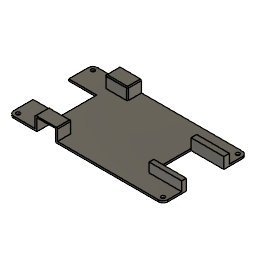
BASE (Autodesk Fusion 360 design; units mm, degrees)
Autodesk Fusion 360 part; units mm, degrees
sketch "Sketch1" plane through (0, 0, 0) normal (0, 0, 1) x (1, 0, 0)
  line L0 (0, 0) -> (165, 0)
  line L1 (165, 0) -> (165, 90)
  line L2 (165, 90) -> (0, 90)
  line L3 (0, 90) -> (0, 0)
  dimension "d1" = 165
  dimension "d2" = 90
  constraint horizontal L0
  constraint vertical L1
  constraint horizontal L2
  constraint vertical L3
  constraint coincident L0.start L3.end
  measures "d1" distance of L0.start L0.end
  measures "d2" distance of L0.start L2.end
extrude "Extrude1" add sketch "Sketch1" along normal blind 3
fillet "Fillet1" radius 5 1 edges at (0, 0, 1.5)
fillet "Fillet1" radius 5 3 edges at (0, 90, 1.5) (165, 90, 1.5) (165, 0, 1.5)
sketch "Sketch4" plane through (0, 0, 3) normal (0, 0, 1) x (-1, 0, 0)
  arc A0 (-160, 0) -> (-165, -5) centre (-160, -5) ccw
  line L0 (-165, -5) -> (-165, -85)
  arc A1 (-165, -85) -> (-160, -90) centre (-160, -85) ccw
  line L1 (-160, -90) -> (-5, -90)
  arc A2 (-5, -90) -> (0, -85) centre (-5, -85) ccw
  line L2 (0, -85) -> (0, -5)
  arc A3 (0, -5) -> (-5, 0) centre (-5, -5) ccw
  line L3 (-5, 0) -> (-160, 0)
  line L4 (-30, -90) -> (-50, -90)
  line L5 (-50, -90) -> (-50, -77)
  line L6 (-50, -77) -> (-30, -77)
  line L7 (-30, -77) -> (-30, -90)
  line L8 (-30, 0) -> (-50, 0)
  line L9 (-50, 0) -> (-50, -13)
  line L10 (-50, -13) -> (-30, -13)
  line L11 (-30, -13) -> (-30, 0)
  dimension "d9" = 20
  dimension "d10" = 13
  dimension "d11" = 20
  dimension "d12" = 13
  constraint horizontal L4
  constraint vertical L5
  constraint horizontal L6
  constraint vertical L7
  constraint coincident L1 L4.start
  constraint horizontal L8
  constraint vertical L9
  constraint horizontal L10
  constraint vertical L11
  constraint coincident L3 L8.start
  measures "d9" distance of L4.start L4.end
  measures "d10" distance of L4.start L6.end
  measures "d11" distance of L8.start L8.end
  measures "d12" distance of L8.start L10.end
extrude "Extrude2" cut sketch "Sketch4" against normal blind 3 contours L3 L8 L9 L10 L11 | L1 L4 L5 L6 L7
sketch "Sketch5" plane through (0, 0, 3) normal (0, 0, 1) x (-1, 0, 0)
  line L0 (-30, -77) -> (-30, -90)
  line L1 (-30, -90) -> (-5, -90)
  arc A0 (-5, -90) -> (0, -85) centre (-5, -85) ccw
  line L2 (0, -85) -> (0, -5)
  arc A1 (0, -5) -> (-5, 0) centre (-5, -5) ccw
  line L3 (-5, 0) -> (-30, 0)
  line L4 (-30, 0) -> (-30, -13)
  line L5 (-30, -13) -> (-50, -13)
  line L6 (-50, -13) -> (-50, 0)
  line L7 (-50, 0) -> (-160, 0)
  arc A2 (-160, 0) -> (-165, -5) centre (-160, -5) ccw
  line L8 (-165, -5) -> (-165, -85)
  arc A3 (-165, -85) -> (-160, -90) centre (-160, -85) ccw
  line L9 (-160, -90) -> (-50, -90)
  line L10 (-50, -90) -> (-50, -77)
  line L11 (-50, -77) -> (-30, -77)
  circle A4 centre (-120, -45) radius 35
  dimension "d41" = 70
  measures "d41" diameter of A4
sketch "Sketch6" plane through (0, 0, 3) normal (0, 0, 1) x (-1, 0, 0)
  line L0 (-30, -77) -> (-30, -90)
  line L1 (-30, -90) -> (-5, -90)
  arc A0 (-5, -90) -> (0, -85) centre (-5, -85) ccw
  line L2 (0, -85) -> (0, -5)
  arc A1 (0, -5) -> (-5, 0) centre (-5, -5) ccw
  line L3 (-5, 0) -> (-30, 0)
  line L4 (-30, 0) -> (-30, -13)
  line L5 (-30, -13) -> (-50, -13)
  line L6 (-50, -13) -> (-50, 0)
  line L7 (-50, 0) -> (-160, 0)
  arc A2 (-160, 0) -> (-165, -5) centre (-160, -5) ccw
  line L8 (-165, -5) -> (-165, -85)
  arc A3 (-165, -85) -> (-160, -90) centre (-160, -85) ccw
  line L9 (-160, -90) -> (-50, -90)
  line L10 (-50, -90) -> (-50, -77)
  line L11 (-50, -77) -> (-30, -77)
  line L12 (-5, -45) -> (-5, -60)
  line L13 (-5, -60) -> (-20, -60)
  line L14 (-20, -60) -> (-20, -30)
  line L15 (-20, -30) -> (-5, -30)
  line L16 (-5, -30) -> (-5, -45)
  line L17 (0, -65) -> (-25, -65)
  line L18 (-25, -65) -> (-25, -25)
  line L19 (-25, -25) -> (0, -25)
  line L20 (0, -25) -> (0, -65)
  dimension "d20" = 15
  dimension "d21" = 15
  constraint parallel L2 L12
  constraint perpendicular L2 L13
  constraint perpendicular L13 L14
  constraint perpendicular L2 L15
  constraint perpendicular L15 L16
  constraint horizontal L17
  constraint vertical L18
  constraint horizontal L19
  constraint vertical L20
  constraint coincident L2 L17.start
  measures "d20" distance of L12.start L12.end
  measures "d21" distance of L12.end L13.end
extrude "Extrude4" add sketch "Sketch6" along normal blind 15 contours L2 L17 L18 L19 L20
sketch "Sketch7" plane through (0, 0, 3) normal (0, 0, 1) x (-1, 0, 0)
  line L0 (0, -65) -> (-25, -65)
  line L1 (-25, -65) -> (-25, -25)
  line L2 (-25, -25) -> (0, -25)
  line L3 (0, -25) -> (0, -5)
  arc A0 (0, -5) -> (-5, 0) centre (-5, -5) ccw
  line L4 (-5, 0) -> (-30, 0)
  line L5 (-30, 0) -> (-30, -13)
  line L6 (-30, -13) -> (-50, -13)
  line L7 (-50, -13) -> (-50, 0)
  line L8 (-50, 0) -> (-160, 0)
  arc A1 (-160, 0) -> (-165, -5) centre (-160, -5) ccw
  line L9 (-165, -5) -> (-165, -85)
  arc A2 (-165, -85) -> (-160, -90) centre (-160, -85) ccw
  line L10 (-160, -90) -> (-50, -90)
  line L11 (-50, -90) -> (-50, -77)
  line L12 (-50, -77) -> (-30, -77)
  line L13 (-30, -77) -> (-30, -90)
  line L14 (-30, -90) -> (-5, -90)
  arc A3 (-5, -90) -> (0, -85) centre (-5, -85) ccw
  line L15 (0, -85) -> (0, -65)
  line L16 (-25, 0) -> (-55, 0)
  line L17 (-55, 0) -> (-55, -15)
  line L18 (-55, -15) -> (-25, -15)
  line L19 (-25, -15) -> (-25, 0)
  line L20 (-25, -90) -> (-55, -90)
  line L21 (-55, -90) -> (-55, -75)
  line L22 (-55, -75) -> (-25, -75)
  line L23 (-25, -75) -> (-25, -90)
  constraint horizontal L16
  constraint vertical L17
  constraint horizontal L18
  constraint vertical L19
  constraint coincident L4 L16.start
  constraint horizontal L20
  constraint vertical L21
  constraint horizontal L22
  constraint vertical L23
  constraint coincident L14 L20.start
extrude "Extrude5" add sketch "Sketch7" along normal blind 10 contours L10 L11 L12 L13 L14 L20 L21 L22 L23 | L4 L5 L6 L7 L8 L16 L17 L18 L19
sketch "Sketch9" plane through (0, 0, 13) normal (0, 0, 1) x (-1, 0, 0)
  line L0 (-50, -90) -> (-50, -77)
  line L1 (-50, -77) -> (-30, -77)
  line L2 (-30, -77) -> (-30, -90)
  line L3 (-30, -90) -> (-25, -90)
  line L4 (-25, -90) -> (-25, -75)
  line L5 (-25, -75) -> (-55, -75)
  line L6 (-55, -75) -> (-55, -90)
  line L7 (-55, -90) -> (-50, -90)
  line L8 (-25, -90) -> (-55, -90)
  line L9 (-55, -90) -> (-55, -75)
  line L10 (-55, -75) -> (-25, -75)
  line L11 (-25, -75) -> (-25, -90)
  constraint horizontal L8
  constraint vertical L9
  constraint horizontal L10
  constraint vertical L11
  constraint coincident L5.end L6.start
  constraint coincident L3.end L4.start
extrude "Extrude6" add sketch "Sketch9" along normal blind 2.5
sketch "Sketch10" plane through (0, 0, 13) normal (0, 0, 1) x (-1, 0, 0)
  line L0 (-25, -15) -> (-25, 0)
  line L1 (-25, 0) -> (-30, 0)
  line L2 (-30, 0) -> (-30, -13)
  line L3 (-30, -13) -> (-50, -13)
  line L4 (-50, -13) -> (-50, 0)
  line L5 (-50, 0) -> (-55, 0)
  line L6 (-55, 0) -> (-55, -15)
  line L7 (-55, -15) -> (-25, -15)
  line L8 (-25, -15) -> (-55, -15)
  line L9 (-55, -15) -> (-55, 0)
  line L10 (-55, 0) -> (-25, 0)
  line L11 (-25, 0) -> (-25, -15)
  constraint horizontal L8
  constraint vertical L9
  constraint horizontal L10
  constraint vertical L11
  constraint coincident L5.end L6.start
  constraint coincident L0.start L7.end
extrude "Extrude7" add sketch "Sketch10" along normal blind 2.5
extrude "Extrude8" cut 1 faces at (10, 40, 3) along direction (0, 0, -1) blind 3
sketch "Sketch11" plane through (0, 0, 3) normal (0, 0, 1) x (-1, 0, 0)
  line L0 (-55, -15) -> (-55, 0)
  line L1 (-55, 0) -> (-160, 0)
  arc A0 (-160, 0) -> (-165, -5) centre (-160, -5) ccw
  line L2 (-165, -5) -> (-165, -85)
  arc A1 (-165, -85) -> (-160, -90) centre (-160, -85) ccw
  line L3 (-160, -90) -> (-55, -90)
  line L4 (-55, -90) -> (-55, -75)
  line L5 (-55, -75) -> (-25, -75)
  line L6 (-25, -75) -> (-25, -90)
  line L7 (-25, -90) -> (-5, -90)
  arc A2 (-5, -90) -> (0, -85) centre (-5, -85) ccw
  line L8 (0, -85) -> (0, -65)
  line L9 (0, -65) -> (-25, -65)
  line L10 (-25, -65) -> (-25, -25)
  line L11 (-25, -25) -> (0, -25)
  arc A3 (0, -5) -> (-5, 0) centre (-5, -5) ccw
  line L12 (-5, 0) -> (-25, 0)
  line L13 (-25, 0) -> (-25, -15)
  line L14 (-25, -15) -> (-55, -15)
  circle A4 centre (-5, -85) radius 2
  circle A5 centre (-5, -5) radius 2
  circle A6 centre (-160, -5) radius 2
  circle A7 centre (-160, -85) radius 2
  line L15 (0, -25) -> (0, -5)
  dimension "d42" = 4
  dimension "d43" = 4
  dimension "d44" = 4
  dimension "d45" = 4
  constraint concentric A2 A4
  constraint concentric A3 A5
  constraint concentric A0 A6
  constraint concentric A1 A7
  measures "d42" diameter of A4
  measures "d43" diameter of A5
  measures "d44" diameter of A6
  measures "d45" diameter of A7
extrude "Extrude9" cut sketch "Sketch11" against normal blind 3 contours A4 | A5 | A6 | A7
extrude "Extrude10" cut 1 faces at (43.3333, 81.3333, 13) along direction (0, 0, 1) blind 1
extrude "Extrude11" cut 1 faces at (43.3333, 4.3333, 13) along direction (0, 0, 1) blind 1
extrude "Extrude12" cut 2 faces at (25, 10, 11.3333) (25, 85, 11.3333) along direction (1, 0, 0) blind 3
extrude "Extrude13" cut 1 faces at (55, 5, 11.3333) along direction (-1, 0, 0) blind 3
extrude "Extrude14" cut 1 faces at (55, 80, 11.3333) along direction (-1, 0, 0) blind 3
extrude "Extrude15" cut 1 faces at (122.1997, 55.6667, 0) along direction (0, 0, 1) blind 1
extrude "Extrude16" cut 1 faces at (23.3333, 40, 18) along direction (0, 0, -1) blind 15
sketch "Sketch12" plane through (0, 0, 1) normal (0, 0, -1) x (1, 0, 0)
  circle A0 centre (5, -5) radius 2
  circle A1 centre (160, -85) radius 2
  circle A2 centre (5, -85) radius 2
  circle A3 centre (160, -5) radius 2
  line L0 (20, -60) -> (5, -60)
  line L1 (5, -60) -> (5, -30)
  line L2 (5, -30) -> (20, -30)
  line L3 (20, -30) -> (20, -60)
  line L4 (30, -90) -> (30, -77)
  line L5 (30, -77) -> (50, -77)
  line L6 (50, -77) -> (50, -90)
  line L7 (50, -90) -> (160, -90)
  arc A4 (160, -90) -> (165, -85) centre (160, -85) ccw
  line L8 (165, -85) -> (165, -5)
  arc A5 (165, -5) -> (160, 0) centre (160, -5) ccw
  line L9 (160, 0) -> (50, 0)
  line L10 (50, 0) -> (50, -13)
  line L11 (50, -13) -> (30, -13)
  line L12 (30, -13) -> (30, 0)
  line L13 (30, 0) -> (5, 0)
  arc A6 (5, 0) -> (0, -5) centre (5, -5) ccw
  line L14 (0, -5) -> (0, -85)
  arc A7 (0, -85) -> (5, -90) centre (5, -85) ccw
  line L15 (5, -90) -> (30, -90)
  line L16 (130, -65) -> (165, -65)
  line L17 (165, -65) -> (165, -25)
  line L18 (165, -25) -> (130, -25)
  line L19 (130, -25) -> (130, -65)
  constraint horizontal L16
  constraint vertical L17
  constraint horizontal L18
  constraint vertical L19
  constraint coincident L8 L17.end
extrude "Extrude17" cut sketch "Sketch12" against normal blind 2 contours L8 L16 L17 L18 L19
sketch "Sketch13" plane through (0, 0, 3) normal (0, 0, 1) x (-1, 0, 0)
  line L0 (-165, -25) -> (-130, -25)
  line L1 (-130, -25) -> (-130, -65)
  line L2 (-130, -65) -> (-165, -65)
  line L3 (-165, -65) -> (-165, -85)
  arc A0 (-165, -85) -> (-160, -90) centre (-160, -85) ccw
  line L4 (-160, -90) -> (-52, -90)
  line L5 (-52, -90) -> (-52, -75)
  line L6 (-52, -75) -> (-28, -75)
  line L7 (-28, -75) -> (-28, -90)
  line L8 (-28, -90) -> (-5, -90)
  arc A1 (-5, -90) -> (0, -85) centre (-5, -85) ccw
  line L9 (0, -85) -> (0, -5)
  arc A2 (0, -5) -> (-5, 0) centre (-5, -5) ccw
  line L10 (-5, 0) -> (-28, 0)
  line L11 (-28, 0) -> (-28, -15)
  line L12 (-28, -15) -> (-52, -15)
  line L13 (-52, -15) -> (-52, 0)
  line L14 (-52, 0) -> (-160, 0)
  arc A3 (-160, 0) -> (-165, -5) centre (-160, -5) ccw
  line L15 (-165, -5) -> (-165, -25)
  circle A4 centre (-160, -5) radius 2
  circle A5 centre (-5, -85) radius 2
  circle A6 centre (-160, -85) radius 2
  circle A7 centre (-5, -5) radius 2
  line L16 (-20, -30) -> (-5, -30)
  line L17 (-5, -30) -> (-5, -60)
  line L18 (-5, -60) -> (-20, -60)
  line L19 (-20, -60) -> (-20, -30)
  line L20 (-165, -20) -> (-130, -20)
  line L21 (-130, -20) -> (-130, -71)
  line L22 (-130, -71) -> (-165, -71)
  line L23 (-165, -71) -> (-165, -20)
  constraint horizontal L20
  constraint vertical L21
  constraint horizontal L22
  constraint vertical L23
  constraint coincident L15 L20.start
extrude "Extrude18" add sketch "Sketch13" along normal blind 10 contours L0 L15 L20 L21 L23 | L2 L3 L21 L22 L23
fillet "Fillet7" radius 1 10 edges at (52, 7.5, 15.5) (28, 7.5, 15.5) (40, 15, 15.5) (52, 82.5, 15.5) (40, 75, 15.5) (28, 82.5, 15.5) (52, 75, 9.25) (28, 75, 9.25) (52, 15, 9.25) (28, 15, 9.25)
sketch "Sketch14" plane through (0, 0, 3) normal (0, 0, 1) x (-1, 0, 0)
  arc A0 (-165, -85) -> (-160, -90) centre (-160, -85) ccw
  line L0 (-160, -90) -> (-52, -90)
  line L1 (-52, -90) -> (-52, -76)
  arc A1 (-51, -75) -> (-52, -76) centre (-51, -76) ccw
  line L2 (-51, -75) -> (-29, -75)
  arc A2 (-28, -76) -> (-29, -75) centre (-29, -76) ccw
  line L3 (-28, -76) -> (-28, -90)
  line L4 (-28, -90) -> (-5, -90)
  arc A3 (-5, -90) -> (0, -85) centre (-5, -85) ccw
  line L5 (0, -85) -> (0, -5)
  arc A4 (0, -5) -> (-5, 0) centre (-5, -5) ccw
  line L6 (-5, 0) -> (-28, 0)
  line L7 (-28, 0) -> (-28, -14)
  arc A5 (-29, -15) -> (-28, -14) centre (-29, -14) ccw
  line L8 (-29, -15) -> (-51, -15)
  arc A6 (-52, -14) -> (-51, -15) centre (-51, -14) ccw
  line L9 (-52, -14) -> (-52, 0)
  line L10 (-52, 0) -> (-160, 0)
  arc A7 (-160, 0) -> (-165, -5) centre (-160, -5) ccw
  line L11 (-165, -20) -> (-130, -20)
  line L12 (-130, -25) -> (-130, -65)
  line L13 (-130, -71) -> (-165, -71)
  circle A8 centre (-160, -5) radius 2
  circle A9 centre (-5, -85) radius 2
  circle A10 centre (-160, -85) radius 2
  circle A11 centre (-5, -5) radius 2
  line L14 (-20, -30) -> (-5, -30)
  line L15 (-5, -30) -> (-5, -60)
  line L16 (-5, -60) -> (-20, -60)
  line L17 (-20, -60) -> (-20, -30)
  line L18 (0, -64) -> (-30, -64)
  line L19 (-30, -64) -> (-30, -26)
  line L20 (-30, -26) -> (0, -26)
  line L21 (0, -26) -> (0, -64)
  line L22 (-165, -71) -> (-165, -85)
  line L23 (-165, -5) -> (-165, -20)
  line L24 (-130, -20) -> (-130, -25)
  line L25 (-130, -65) -> (-130, -71)
  dimension "d70" = 30
  dimension "d71" = 38
  constraint horizontal L18
  constraint vertical L19
  constraint horizontal L20
  constraint vertical L21
  constraint coincident L5 L18.start
  measures "d70" distance of L18.start L18.end
  measures "d71" distance of L18.start L20.end
extrude "Extrude19" cut sketch "Sketch14" against normal blind 2 contours L5 L18 L19 L20 L21
